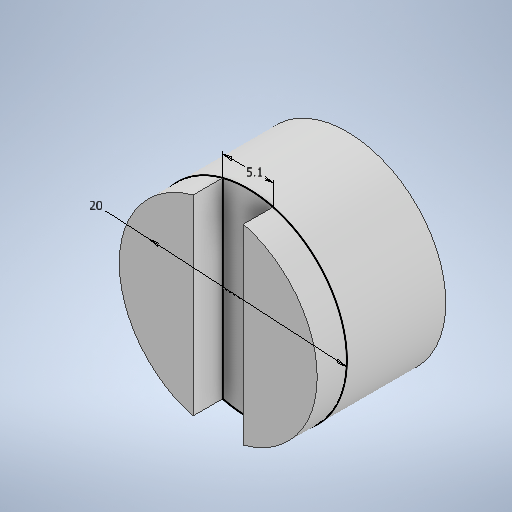
# Autodesk Inventor part: ToolMount
Saved by Autodesk Inventor 2025.3 (Build 293356030, 356C)
## iProperties
Created: 2025-10-10
Part Number: ToolMount
Material: Generic
Document SubType Name: Modeling
Designer: tvoko
Density: 1 g/cm^3
Appearance: Default
Author: tvoko
Autodesk Inventor part; units mm, degrees
ref_plane "YZ Plane" through (0, 0, 0) normal (1, 0, 0) x (0, 1, 0)
ref_plane "XZ Plane" through (0, 0, 0) normal (0, 1, 0) x (-1, 0, 0)
ref_plane "XY Plane" through (0, 0, 0) normal (0, 0, 1) x (1, 0, 0)
sketch "Sketch2" plane through (0, 0, 0) normal (0, 0, 1) x (1, 0, 0)
  circle A0 centre (0, 0) radius 10
  line L0 (-2.55, 0) -> (2.55, 0) construction
  line L1 (-2.55, 9.6694) -> (-2.55, -9.6694)
  line L2 (2.55, 9.6694) -> (2.55, -9.6694)
  dimension "d0" = 5.1
  dimension "d1" = 20
  constraints: 6 end point, 4 point on circle, 3 midpoint, 2 coincident, 1 centre point, 1 horizontal
  measures "d0" distance between parallel lines of L2 L1
  measures "d1" diameter of A0
extrude "Extrusion1" add sketch "Sketch2" against normal blind 10
extrude "Extrusion2" add sketch "Sketch2" along normal blind 3 contours A0 L2 | L1 A0
body "Solid1"
